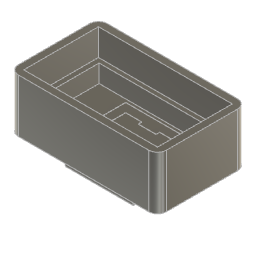
Master Arm AA AG v11 (Autodesk Fusion 360 design; units mm, degrees)
Autodesk Fusion 360 part; units mm, degrees
(part 1 of 6)
sketch "Master Arm Legend Plate" plane through (-25, -275, 0) normal (0, 0, 1) x (1, 0, 0)
  line L0 (41.275, 261.179028) -> (41.521944, 261.14375)
  line L1 (42.545, 261.955139) -> (42.545, 262.202083)
  line L2 (41.521944, 261.14375) -> (41.839444, 261.179028)
  line L3 (8.678333, 226.924305) -> (8.713611, 226.994861)
  line L4 (8.713611, 226.994861) -> (8.748889, 227.100694)
  line L5 (6.385278, 226.85375) -> (8.396111, 226.85375)
  line L6 (32.984722, 286.190972) -> (33.196389, 286.120417)
  line L7 (33.196389, 286.120417) -> (33.443333, 286.085139)
  line L8 (42.051111, 264.424583) -> (41.874722, 264.671528)
  line L9 (23.459722, 289.295417) -> (21.448889, 289.295417)
  line L10 (21.448889, 289.295417) -> (21.448889, 288.201805)
  line L11 (21.448889, 288.201805) -> (22.895278, 288.201805)
  line L12 (37.958889, 291.059305) -> (35.771667, 291.059305)
  line L13 (35.595278, 285.555972) -> (35.489444, 285.59125)
  line L14 (31.220833, 295.222083) -> (31.291389, 295.11625)
  line L15 (30.056667, 253.594305) -> (30.127222, 253.594305)
  line L16 (35.771667, 227.241805) -> (35.771667, 227.100694)
  line L17 (43.991389, 295.821805) -> (43.991389, 295.186805)
  line L18 (25.646944, 224.878194) -> (25.752778, 224.984028)
  line L19 (42.721389, 272.503194) -> (42.721389, 272.397361)
  line L20 (42.721389, 272.397361) -> (42.686111, 272.326805)
  line L21 (42.686111, 272.326805) -> (42.580278, 272.25625)
  line L22 (42.580278, 272.25625) -> (42.474444, 272.25625)
  line L23 (42.474444, 272.25625) -> (42.403889, 272.25625)
  line L24 (42.403889, 272.25625) -> (42.333333, 272.291528)
  line L25 (42.333333, 272.291528) -> (42.262778, 272.362083)
  line L26 (42.262778, 272.362083) -> (42.2275, 272.432639)
  line L27 (42.2275, 272.432639) -> (42.051111, 272.961805)
  line L28 (42.051111, 272.961805) -> (40.604722, 272.961805)
  line L29 (40.604722, 272.961805) -> (40.463611, 272.397361)
  line L30 (40.463611, 272.397361) -> (40.428333, 272.326805)
  line L31 (40.428333, 272.326805) -> (40.393056, 272.291528)
  line L32 (40.393056, 272.291528) -> (40.287222, 272.25625)
  line L33 (40.287222, 272.25625) -> (40.216667, 272.25625)
  line L34 (40.216667, 272.25625) -> (40.040278, 272.291528)
  line L35 (40.040278, 272.291528) -> (39.969722, 272.362083)
  line L36 (39.969722, 272.362083) -> (39.934444, 272.467917)
  line L37 (39.934444, 272.467917) -> (39.969722, 272.57375)
  line L38 (39.969722, 272.57375) -> (40.005, 272.679583)
  line L39 (40.005, 272.679583) -> (41.063333, 276.313194)
  line L40 (41.063333, 276.313194) -> (41.098611, 276.38375)
  line L41 (41.098611, 276.38375) -> (41.133889, 276.454305)
  line L42 (41.133889, 276.454305) -> (41.239722, 276.489583)
  line L43 (41.239722, 276.489583) -> (41.345556, 276.489583)
  line L44 (41.345556, 276.489583) -> (41.416111, 276.489583)
  line L45 (41.416111, 276.489583) -> (41.486667, 276.454305)
  line L46 (41.486667, 276.454305) -> (41.557222, 276.348472)
  line L47 (41.557222, 276.348472) -> (41.5925, 276.242639)
  line L48 (41.5925, 276.242639) -> (42.686111, 272.644305)
  line L49 (42.686111, 272.644305) -> (42.721389, 272.57375)
  line L50 (42.721389, 272.57375) -> (42.721389, 272.503194)
  line L51 (33.196389, 241.14125) -> (33.161111, 241.77625)
  line L52 (33.161111, 241.77625) -> (33.090556, 242.375972)
  line L53 (33.090556, 242.375972) -> (32.949444, 243.010972)
  line L54 (32.949444, 243.010972) -> (32.737778, 243.575417)
  line L55 (32.737778, 243.575417) -> (32.455556, 244.139861)
  line L56 (32.455556, 244.139861) -> (32.138056, 244.669028)
  line L57 (32.138056, 244.669028) -> (31.75, 245.198194)
  line L58 (31.75, 245.198194) -> (31.361944, 245.656805)
  line L59 (31.361944, 245.656805) -> (30.868056, 246.080139)
  line L60 (30.868056, 246.080139) -> (30.374167, 246.432917)
  line L61 (30.374167, 246.432917) -> (29.845, 246.750417)
  line L62 (29.845, 246.750417) -> (29.280556, 247.032639)
  line L63 (29.280556, 247.032639) -> (28.716111, 247.244305)
  line L64 (28.716111, 247.244305) -> (28.081111, 247.385417)
  line L65 (28.081111, 247.385417) -> (27.481389, 247.455972)
  line L66 (27.481389, 247.455972) -> (26.846389, 247.49125)
  line L67 (26.846389, 247.49125) -> (26.246667, 247.455972)
  line L68 (26.246667, 247.455972) -> (25.611667, 247.385417)
  line L69 (25.611667, 247.385417) -> (25.011944, 247.244305)
  line L70 (25.011944, 247.244305) -> (24.412222, 247.032639)
  line L71 (24.412222, 247.032639) -> (23.847778, 246.750417)
  line L72 (23.847778, 246.750417) -> (23.318611, 246.432917)
  line L73 (23.318611, 246.432917) -> (22.824722, 246.080139)
  line L74 (22.824722, 246.080139) -> (22.366111, 245.656805)
  line L75 (22.366111, 245.656805) -> (21.942778, 245.198194)
  line L76 (21.942778, 245.198194) -> (21.59, 244.669028)
  line L77 (21.59, 244.669028) -> (21.2725, 244.139861)
  line L78 (21.2725, 244.139861) -> (20.990278, 243.575417)
  line L79 (20.990278, 243.575417) -> (20.778611, 243.010972)
  line L80 (20.778611, 243.010972) -> (20.6375, 242.375972)
  line L81 (20.6375, 242.375972) -> (20.531667, 241.77625)
  line L82 (20.531667, 241.77625) -> (20.496389, 241.14125)
  line L83 (20.496389, 241.14125) -> (20.531667, 240.541528)
  line L84 (20.531667, 240.541528) -> (20.6375, 239.906528)
  line L85 (20.6375, 239.906528) -> (20.778611, 239.306805)
  line L86 (20.778611, 239.306805) -> (20.990278, 238.707083)
  line L87 (20.990278, 238.707083) -> (21.2725, 238.177917)
  line L88 (21.2725, 238.177917) -> (21.59, 237.613472)
  line L89 (21.59, 237.613472) -> (21.942778, 237.119583)
  line L90 (21.942778, 237.119583) -> (22.366111, 236.660972)
  line L91 (22.366111, 236.660972) -> (22.824722, 236.237639)
  line L92 (22.824722, 236.237639) -> (23.318611, 235.884861)
  line L93 (23.318611, 235.884861) -> (23.847778, 235.567361)
  line L94 (23.847778, 235.567361) -> (24.412222, 235.285139)
  line L95 (24.412222, 235.285139) -> (25.011944, 235.073472)
  line L96 (25.011944, 235.073472) -> (25.611667, 234.932361)
  line L97 (25.611667, 234.932361) -> (26.246667, 234.826528)
  line L98 (26.246667, 234.826528) -> (26.846389, 234.79125)
  line L99 (26.846389, 234.79125) -> (27.481389, 234.826528)
  line L100 (27.481389, 234.826528) -> (28.081111, 234.932361)
  line L101 (28.081111, 234.932361) -> (28.716111, 235.073472)
  line L102 (28.716111, 235.073472) -> (29.280556, 235.285139)
  line L103 (29.280556, 235.285139) -> (29.845, 235.567361)
  line L104 (29.845, 235.567361) -> (30.374167, 235.884861)
  line L105 (30.374167, 235.884861) -> (30.868056, 236.237639)
  line L106 (30.868056, 236.237639) -> (31.361944, 236.660972)
  line L107 (31.361944, 236.660972) -> (31.75, 237.119583)
  line L108 (31.75, 237.119583) -> (32.138056, 237.613472)
  line L109 (32.138056, 237.613472) -> (32.455556, 238.177917)
  line L110 (32.455556, 238.177917) -> (32.737778, 238.707083)
  line L111 (32.737778, 238.707083) -> (32.949444, 239.306805)
  line L112 (32.949444, 239.306805) -> (33.090556, 239.906528)
  line L113 (33.090556, 239.906528) -> (33.161111, 240.541528)
  line L114 (33.161111, 240.541528) -> (33.196389, 241.14125)
  line L115 (33.831389, 294.728194) -> (34.043056, 294.587083)
  line L116 (10.089444, 235.602639) -> (10.442222, 235.461528)
  line L117 (10.442222, 235.461528) -> (10.724444, 235.249861)
  line L118 (30.868056, 230.381528) -> (30.938611, 230.381528)
  line L119 (30.938611, 230.381528) -> (31.044444, 230.416805)
  line L120 (31.044444, 230.416805) -> (31.079722, 230.416805)
  line L121 (21.942778, 225.513194) -> (22.013333, 225.548472)
  line L122 (18.273889, 226.85375) -> (18.485556, 226.85375)
  line L123 (18.485556, 226.85375) -> (18.626667, 226.783194)
  line L124 (38.4175, 253.20625) -> (38.452778, 253.170972)
  line L125 (32.490833, 291.165139) -> (32.526111, 291.376805)
  line L126 (20.919722, 285.90875) -> (20.919722, 289.471805)
  line L127 (20.919722, 289.471805) -> (20.919722, 289.612917)
  line L128 (20.919722, 289.612917) -> (20.955, 289.71875)
  line L129 (41.733611, 263.542639) -> (41.627778, 263.542639)
  line L130 (41.627778, 263.542639) -> (41.521944, 263.507361)
  line L131 (40.040278, 253.100417) -> (40.110833, 253.170972)
  line L132 (41.980556, 265.27125) -> (42.192222, 265.130139)
  line L133 (42.509722, 264.354028) -> (42.403889, 264.283472)
  line L134 (41.768889, 261.708194) -> (41.874722, 261.77875)
  line L135 (39.828611, 231.404583) -> (39.793333, 231.686805)
  line L136 (39.793333, 231.686805) -> (39.722778, 231.863194)
  line L137 (39.722778, 231.863194) -> (39.581667, 231.969028)
  line L138 (39.581667, 231.969028) -> (39.511111, 232.039583)
  line L139 (39.511111, 232.039583) -> (39.37, 232.039583)
  line L140 (39.37, 232.039583) -> (38.735, 232.039583)
  line L141 (38.735, 232.039583) -> (38.735, 230.769583)
  line L142 (38.735, 230.769583) -> (39.334722, 230.769583)
  line L143 (39.334722, 230.769583) -> (39.475833, 230.769583)
  line L144 (39.475833, 230.769583) -> (39.581667, 230.840139)
  line L145 (39.581667, 230.840139) -> (39.652222, 230.910694)
  line L146 (39.652222, 230.910694) -> (39.793333, 231.087083)
  line L147 (39.793333, 231.087083) -> (39.828611, 231.404583)
  line L148 (42.474444, 263.507361) -> (42.545, 263.36625)
  line L149 (14.2875, 290.177361) -> (14.075833, 289.824583)
  line L150 (14.075833, 289.824583) -> (13.97, 289.471805)
  line L151 (9.913056, 223.255417) -> (9.877778, 223.220139)
  line L152 (38.946667, 276.807083) -> (39.017222, 276.807083)
  line L153 (34.572222, 289.189583) -> (34.6075, 289.08375)
  line L154 (34.6075, 289.08375) -> (34.642778, 288.977917)
  line L155 (21.131389, 285.555972) -> (21.025556, 285.626528)
  line L156 (21.025556, 285.626528) -> (20.919722, 285.767639)
  line L157 (20.919722, 285.767639) -> (20.919722, 285.90875)
  line L158 (31.361944, 245.656805) -> (30.868056, 246.080139)
  line L159 (30.868056, 246.080139) -> (30.374167, 246.432917)
  line L160 (41.310278, 261.708194) -> (41.557222, 261.672917)
  line L161 (25.893889, 225.019305) -> (26.035, 224.984028)
  line L162 (42.721389, 272.397361) -> (42.721389, 272.503194)
  line L163 (35.806944, 261.320139) -> (35.842222, 261.249583)
  line L164 (38.311667, 244.245694) -> (38.276389, 243.928194)
  line L165 (34.536944, 291.059305) -> (34.642778, 291.094583)
  line L166 (31.291389, 295.010417) -> (31.291389, 291.341528)
  line L167 (32.243889, 279.135417) -> (32.208611, 279.452917)
  line L168 (28.363333, 223.714028) -> (28.575, 224.066805)
  line L169 (25.611667, 224.63125) -> (25.682222, 224.207917)
  line L170 (25.682222, 224.207917) -> (25.893889, 223.784583)
  line L171 (32.102778, 245.939028) -> (31.644167, 246.397639)
  line L172 (31.644167, 246.397639) -> (31.150278, 246.820972)
  line L173 (42.474444, 264.777361) -> (42.580278, 264.565694)
  line L174 (31.115, 230.557917) -> (31.115, 230.628472)
  line L175 (28.716111, 230.452083) -> (28.716111, 230.557917)
  line L176 (27.6225, 230.381528) -> (28.433889, 230.381528)
  line L177 (27.6225, 228.970417) -> (27.6225, 230.381528)
  line L178 (14.851944, 290.741805) -> (14.534444, 290.494861)
  line L179 (14.534444, 290.494861) -> (14.2875, 290.177361)
  line L180 (21.2725, 244.139861) -> (21.59, 244.669028)
  line L181 (27.269722, 294.939861) -> (27.305, 295.080972)
  line L182 (24.765, 289.471805) -> (24.729722, 289.577639)
  line L183 (39.123056, 265.694583) -> (39.0525, 265.624028)
  line L184 (24.729722, 289.577639) -> (24.765, 289.648194)
  line L185 (32.490833, 286.755417) -> (32.7025, 286.437917)
  line L186 (32.7025, 286.437917) -> (32.984722, 286.190972)
  line L187 (38.241111, 236.555139) -> (38.382222, 236.625694)
  line L188 (40.3225, 236.308194) -> (40.287222, 236.237639)
  line L189 (38.4175, 228.75875) -> (38.488056, 228.723472)
  line L190 (38.276389, 229.040972) -> (38.276389, 228.899861)
  line L191 (19.05, 226.148194) -> (19.014722, 226.324583)
  line L192 (19.014722, 226.324583) -> (18.944167, 226.500972)
  line L193 (18.944167, 226.500972) -> (18.803056, 226.677361)
  line L194 (18.803056, 226.677361) -> (18.626667, 226.783194)
  line L195 (18.626667, 226.783194) -> (18.485556, 226.85375)
  line L196 (18.485556, 226.85375) -> (18.273889, 226.85375)
  line L197 (18.273889, 226.85375) -> (17.321389, 226.85375)
  line L198 (17.321389, 226.85375) -> (17.321389, 225.407361)
  line L199 (17.321389, 225.407361) -> (18.238611, 225.407361)
  line L200 (18.238611, 225.407361) -> (18.415, 225.442639)
  line L201 (18.415, 225.442639) -> (18.626667, 225.477917)
  line L202 (18.626667, 225.477917) -> (18.803056, 225.58375)
  line L203 (18.803056, 225.58375) -> (18.908889, 225.724861)
  line L204 (18.908889, 225.724861) -> (19.014722, 225.936528)
  line L205 (19.014722, 225.936528) -> (19.05, 226.148194)
  line L206 (38.664444, 236.167083) -> (40.040278, 236.167083)
  line L207 (38.664444, 235.214583) -> (38.664444, 236.167083)
  line L208 (39.6875, 235.214583) -> (38.664444, 235.214583)
  line L209 (39.934444, 235.002917) -> (39.934444, 235.073472)
  line L210 (21.942778, 225.019305) -> (21.872222, 225.054583)
  line L211 (38.735, 243.928194) -> (38.770278, 243.751805)
  line L212 (34.642778, 287.637361) -> (34.642778, 286.614305)
  line L213 (34.642778, 286.614305) -> (34.6075, 286.367361)
  line L214 (39.0525, 227.382917) -> (39.264167, 227.312361)
  line L215 (39.264167, 227.312361) -> (39.37, 227.241805)
  line L216 (39.228889, 276.419028) -> (39.193611, 276.277917)
  line L217 (27.481389, 232.004305) -> (28.821944, 232.004305)
  line L218 (33.760833, 285.626528) -> (33.408056, 285.555972)
  line L219 (33.408056, 285.555972) -> (33.090556, 285.59125)
  line L220 (29.598056, 293.422917) -> (29.562778, 293.317083)
  line L221 (30.021389, 250.313472) -> (29.986111, 250.34875)
  line L222 (26.246667, 247.455972) -> (26.846389, 247.49125)
  line L223 (26.176111, 223.467083) -> (25.893889, 223.784583)
  line L224 (16.792222, 286.931805) -> (17.109722, 287.108194)
  line L225 (17.109722, 287.108194) -> (17.427222, 287.284583)
  line L226 (37.817778, 287.707917) -> (35.806944, 287.707917)
  line L227 (43.991389, 287.390417) -> (43.991389, 282.486805)
  line L228 (20.531667, 240.541528) -> (20.496389, 241.14125)
  line L229 (37.641389, 293.21125) -> (37.394444, 293.175972)
  line L230 (40.428333, 272.326805) -> (40.463611, 272.397361)
  line L231 (39.934444, 272.467917) -> (39.969722, 272.362083)
  line L232 (39.698083, 284.522333) -> (39.334722, 284.885694)
  line L233 (39.405278, 265.624028) -> (39.440556, 265.553472)
  line L234 (40.357778, 240.541528) -> (40.3225, 240.470972)
  line L235 (33.196389, 226.85375) -> (32.984722, 226.889028)
  line L236 (32.984722, 226.889028) -> (32.914167, 226.959583)
  line L237 (9.595556, 227.347639) -> (9.666111, 227.347639)
  line L238 (33.478611, 243.716528) -> (33.231667, 244.31625)
  line L239 (33.231667, 244.31625) -> (32.914167, 244.880694)
  line L240 (37.076944, 272.25625) -> (36.971111, 272.25625)
  line L241 (26.846389, 247.49125) -> (27.481389, 247.455972)
  line L242 (34.360556, 288.695694) -> (34.29, 288.695694)
  line L243 (34.29, 288.695694) -> (34.219444, 288.730972)
  line L244 (30.303611, 250.454583) -> (30.303611, 250.384028)
  line L245 (14.781389, 280.722917) -> (30.656389, 280.722917)
  line L246 (33.831389, 242.446528) -> (33.690278, 243.116805)
  line L247 (33.690278, 243.116805) -> (33.478611, 243.716528)
  line L248 (30.338889, 250.525139) -> (30.303611, 250.454583)
  line L249 (39.264167, 276.665972) -> (39.264167, 276.524861)
  line L250 (34.29, 287.990139) -> (33.655, 287.990139)
  line L251 (40.216667, 249.431528) -> (40.146111, 249.466805)
  line L252 (29.986111, 229.111528) -> (29.986111, 230.381528)
  line L253 (23.106944, 225.336805) -> (23.106944, 225.195694)
  line L254 (14.005278, 288.307639) -> (14.181667, 287.954861)
  line L255 (14.181667, 287.954861) -> (14.393333, 287.637361)
  line L256 (29.598056, 231.757361) -> (29.598056, 231.827917)
  line L257 (22.577778, 235.461528) -> (23.106944, 235.10875)
  line L258 (23.106944, 235.10875) -> (23.671389, 234.79125)
  line L259 (25.893889, 223.784583) -> (25.682222, 224.207917)
  line L260 (28.645556, 224.419583) -> (28.575, 224.066805)
  line L261 (29.562778, 293.317083) -> (29.5275, 293.246528)
  line L262 (37.218056, 272.291528) -> (37.1475, 272.25625)
  line L263 (30.691667, 289.295417) -> (29.845, 289.295417)
  line L264 (32.596667, 288.695694) -> (32.349722, 288.272361)
  line L265 (32.349722, 288.272361) -> (32.279167, 287.990139)
  line L266 (38.241111, 289.71875) -> (38.205833, 289.754028)
  line L267 (38.205833, 289.754028) -> (38.170556, 289.789305)
  line L268 (23.671389, 234.79125) -> (24.271111, 234.509028)
  line L269 (24.271111, 234.509028) -> (24.906111, 234.297361)
  line L270 (36.900556, 272.291528) -> (36.83, 272.397361)
  line L271 (40.357778, 249.466805) -> (40.216667, 249.431528)
  line L272 (27.305, 295.080972) -> (27.340278, 295.186805)
  line L273 (35.806944, 295.292639) -> (37.994167, 295.292639)
  line L274 (37.1475, 272.25625) -> (37.076944, 272.25625)
  line L275 (38.664444, 234.755972) -> (38.664444, 233.344861)
  line L276 (36.971111, 272.25625) -> (36.900556, 272.291528)
  line L277 (34.642778, 287.637361) -> (34.6075, 287.778472)
  line L278 (34.6075, 287.778472) -> (34.536944, 287.919583)
  line L279 (32.984722, 289.154305) -> (32.773056, 288.942639)
  line L280 (32.773056, 288.942639) -> (32.596667, 288.695694)
  line L281 (36.865278, 272.679583) -> (36.865278, 272.714861)
  line L282 (29.421667, 223.184861) -> (29.351111, 223.325972)
  line L283 (39.087778, 237.084305) -> (39.158333, 237.01375)
  line L284 (39.158333, 237.01375) -> (39.264167, 237.01375)
  line L285 (27.551944, 291.059305) -> (27.6225, 291.059305)
  line L286 (16.016111, 223.149583) -> (15.769167, 223.114305)
  line L287 (30.197778, 253.594305) -> (30.268333, 253.559028)
  line L288 (15.980833, 223.643472) -> (15.875, 223.643472)
  line L289 (15.875, 223.643472) -> (15.804444, 223.643472)
  line L290 (29.845, 246.750417) -> (30.374167, 246.432917)
  line L291 (25.611667, 224.63125) -> (25.611667, 224.737083)
  line L292 (27.199167, 231.722083) -> (27.199167, 231.827917)
  line L293 (1.446389, 284.709305) -> (5.150556, 292.999583)
  line L294 (42.580278, 264.565694) -> (42.474444, 264.777361)
  line L295 (19.755556, 241.14125) -> (19.790833, 240.50625)
  line L296 (19.790833, 240.50625) -> (19.861389, 239.835972)
  line L297 (39.581667, 244.422083) -> (39.37, 244.457361)
  line L298 (27.798889, 291.30625) -> (27.798889, 291.200417)
  line L299 (15.769167, 223.114305) -> (16.016111, 223.149583)
  line L300 (40.146111, 244.457361) -> (40.216667, 244.280972)
  line L301 (23.106944, 226.465694) -> (23.106944, 226.53625)
  line L302 (22.577778, 226.430417) -> (22.718889, 226.289305)
  line L303 (22.718889, 226.289305) -> (22.789444, 226.254028)
  line L304 (31.608889, 225.689583) -> (31.644167, 225.58375)
  line L305 (25.153056, 289.754028) -> (25.294167, 289.612917)
  line L306 (31.291389, 280.581805) -> (31.538333, 280.440694)
  line L307 (27.305, 252.88875) -> (27.340278, 252.641805)
  line L308 (8.748889, 227.100694) -> (8.713611, 227.206528)
  line L309 (8.713611, 227.206528) -> (8.678333, 227.277083)
  line L310 (8.678333, 227.277083) -> (8.607778, 227.347639)
  line L311 (29.739167, 228.723472) -> (29.845, 228.723472)
  line L312 (29.598056, 231.757361) -> (29.598056, 228.970417)
  line L313 (29.845, 232.004305) -> (29.739167, 232.004305)
  line L314 (28.716111, 230.628472) -> (28.716111, 230.557917)
  line L315 (35.277778, 273.490972) -> (34.148889, 273.490972)
  line L316 (34.148889, 273.490972) -> (34.713333, 275.325417)
  line L317 (21.59, 244.669028) -> (21.2725, 244.139861)
  line L318 (21.2725, 244.139861) -> (20.990278, 243.575417)
  line L319 (30.868056, 236.237639) -> (30.374167, 235.884861)
  line L320 (9.595556, 227.347639) -> (9.489722, 227.312361)
  line L321 (9.489722, 227.312361) -> (9.454444, 227.241805)
  line L322 (32.173333, 223.537639) -> (32.208611, 223.467083)
  line L323 (33.372778, 287.919583) -> (33.443333, 287.954861)
  line L324 (33.443333, 287.954861) -> (33.549167, 287.990139)
  line L325 (14.322778, 295.821805) -> (19.261667, 295.821805)
  line L326 (17.885833, 281.745972) -> (12.946944, 281.745972)
  line L327 (32.102778, 226.889028) -> (31.996944, 226.85375)
  line L328 (36.583056, 227.312361) -> (36.83, 227.382917)
  line L329 (29.351111, 223.325972) -> (29.315833, 223.467083)
  line L330 (34.219444, 294.234305) -> (34.254722, 294.057917)
  line L331 (33.196389, 241.14125) -> (33.161111, 240.541528)
  line L332 (31.785278, 257.369028) -> (31.538333, 257.157361)
  line L333 (18.626667, 225.477917) -> (18.415, 225.442639)
  line L334 (10.442222, 235.461528) -> (10.089444, 235.602639)
  line L335 (10.089444, 235.602639) -> (9.736667, 235.673194)
  line L336 (9.736667, 235.673194) -> (9.383889, 235.673194)
  line L337 (23.847778, 235.567361) -> (23.318611, 235.884861)
  line L338 (33.161111, 241.77625) -> (33.196389, 241.14125)
  line L339 (37.711944, 293.599305) -> (37.747222, 293.52875)
  line L340 (32.949444, 239.306805) -> (32.737778, 238.707083)
  line L341 (31.467778, 231.722083) -> (31.397222, 231.651528)
  line L342 (34.819167, 265.377083) -> (34.748611, 265.341805)
  line L343 (34.748611, 265.341805) -> (34.678056, 265.27125)
  line L344 (34.678056, 265.27125) -> (34.642778, 265.200694)
  line L345 (39.334722, 295.43375) -> (39.334722, 295.821805)
  line L346 (27.375556, 286.014583) -> (27.446111, 285.944028)
  line L347 (31.891111, 223.643472) -> (31.961667, 223.643472)
  line L348 (38.558611, 249.749028) -> (38.523333, 249.537361)
  line L349 (36.935833, 281.745972) -> (39.698083, 284.522333)
  line L350 (22.013333, 225.019305) -> (22.119167, 225.019305)
  line L351 (38.981944, 265.553472) -> (37.076944, 261.602361)
  line L352 (39.228889, 265.694583) -> (39.123056, 265.694583)
  line L353 (40.463611, 252.959305) -> (40.463611, 253.100417)
  line L354 (40.463611, 253.100417) -> (40.393056, 253.170972)
  line L355 (40.393056, 253.170972) -> (40.3225, 253.20625)
  line L356 (16.016111, 226.889028) -> (16.051389, 226.924305)
  line L357 (28.539722, 227.347639) -> (28.610278, 227.312361)
  line L358 (42.439167, 261.637639) -> (42.545, 261.955139)
  line L359 (29.280556, 251.442361) -> (29.245278, 251.442361)
  line L360 (40.005, 251.93625) -> (39.511111, 250.913194)
  line L361 (18.415, 225.442639) -> (18.238611, 225.407361)
  line L362 (18.626667, 226.783194) -> (18.803056, 226.677361)
  line L363 (8.748889, 223.255417) -> (8.713611, 223.220139)
  line L364 (8.713611, 223.220139) -> (8.643056, 223.149583)
  line L365 (11.006667, 235.038194) -> (10.724444, 235.249861)
  line L366 (10.724444, 235.249861) -> (10.442222, 235.461528)
  line L367 (31.644167, 225.513194) -> (31.608889, 225.372083)
  line L368 (37.676667, 223.396528) -> (37.676667, 223.290694)
  line L369 (37.676667, 226.85375) -> (37.676667, 223.467083)
  line L370 (36.794722, 226.85375) -> (37.676667, 226.85375)
  line L371 (22.154444, 226.818472) -> (22.330833, 226.712639)
  line L372 (22.330833, 226.712639) -> (22.577778, 226.430417)
  line L373 (21.060833, 226.254028) -> (21.237222, 226.500972)
  line L374 (15.522222, 225.689583) -> (15.451667, 225.724861)
  line L375 (15.451667, 225.724861) -> (15.24, 225.760139)
  line L376 (15.204722, 225.26625) -> (15.451667, 225.301528)
  line L377 (29.280556, 235.285139) -> (28.716111, 235.073472)
  line L378 (38.276389, 241.740972) -> (38.205833, 242.164305)
  line L379 (26.740556, 289.754028) -> (26.67, 289.648194)
  line L380 (27.199167, 253.559028) -> (26.916944, 253.594305)
  line L381 (28.645556, 253.488472) -> (28.610278, 253.52375)
  line L382 (43.074167, 218.034306) -> (43.991389, 218.034306)
  line L383 (29.950833, 222.549861) -> (25.435278, 218.034306)
  line L384 (40.781111, 262.590139) -> (40.675278, 262.907639)
  line L385 (30.021389, 234.79125) -> (30.585833, 235.10875)
  line L386 (30.585833, 235.10875) -> (31.150278, 235.461528)
  line L387 (43.991389, 293.740417) -> (43.991389, 288.836805)
  line L388 (32.208611, 289.119028) -> (31.926389, 288.589861)
  line L389 (25.964444, 250.595694) -> (25.964444, 250.454583)
  line L390 (25.964444, 250.454583) -> (25.964444, 250.419305)
  line L391 (16.157222, 223.396528) -> (16.121944, 223.467083)
  line L392 (16.121944, 223.467083) -> (16.086667, 223.537639)
  line L393 (16.086667, 223.537639) -> (15.980833, 223.643472)
  line L394 (39.123056, 241.14125) -> (38.770278, 241.211805)
  line L395 (24.412222, 247.032639) -> (25.011944, 247.244305)
  line L396 (31.785278, 288.13125) -> (31.926389, 288.589861)
  line L397 (31.926389, 288.589861) -> (32.208611, 289.119028)
  line L398 (34.642778, 291.094583) -> (34.748611, 291.165139)
  line L399 (39.334722, 289.08375) -> (43.991389, 293.740417)
  line L400 (24.800278, 289.365972) -> (24.765, 289.471805)
  line L401 (37.747222, 293.317083) -> (37.711944, 293.246528)
  line L402 (27.163889, 289.683472) -> (27.093333, 289.754028)
  line L403 (28.328056, 250.34875) -> (28.292778, 250.384028)
  line L404 (23.318611, 235.884861) -> (22.824722, 236.237639)
  line L405 (35.136667, 265.235972) -> (35.066111, 265.341805)
  line L406 (35.066111, 265.341805) -> (34.995556, 265.377083)
  line L407 (9.383889, 235.673194) -> (9.736667, 235.673194)
  line L408 (9.736667, 235.673194) -> (10.089444, 235.602639)
  line L409 (12.206111, 223.149583) -> (12.135556, 223.184861)
  line L410 (40.781111, 273.490972) -> (41.345556, 275.325417)
  line L411 (24.341667, 252.677083) -> (24.765, 251.265972)
  line L412 (21.872222, 225.054583) -> (21.942778, 225.019305)
  line L413 (21.942778, 225.019305) -> (22.013333, 225.019305)
  line L414 (31.220833, 231.61625) -> (31.326667, 231.61625)
  line L415 (22.965833, 226.289305) -> (22.86, 226.254028)
  line L416 (25.435278, 250.489861) -> (25.435278, 250.560417)
  line L417 (33.513889, 261.355417) -> (33.549167, 261.249583)
  line L418 (13.6525, 280.264305) -> (13.476111, 280.017361)
  line L419 (27.798889, 293.175972) -> (29.21, 293.175972)
  line L420 (27.798889, 291.376805) -> (27.798889, 293.175972)
  line L421 (27.798889, 291.200417) -> (27.798889, 291.30625)
  line L422 (27.798889, 291.30625) -> (27.798889, 291.376805)
  line L423 (28.821944, 231.61625) -> (27.6225, 231.61625)
  line L424 (25.646944, 233.380139) -> (26.317222, 233.309583)
  line L425 (26.317222, 233.309583) -> (27.022778, 233.274305)
  line L426 (27.022778, 233.274305) -> (27.728333, 233.344861)
  line L427 (27.728333, 233.344861) -> (28.398611, 233.450694)
  line L428 (26.3525, 228.723472) -> (26.387778, 228.723472)
  line L429 (26.387778, 228.723472) -> (26.458333, 228.723472)
  line L430 (34.536944, 276.454305) -> (34.466389, 276.38375)
  line L431 (34.466389, 276.38375) -> (34.466389, 276.313194)
  line L432 (29.421667, 251.477639) -> (29.351111, 251.442361)
  line L433 (21.801667, 225.125139) -> (21.766389, 225.26625)
  line L434 (38.664444, 242.199583) -> (38.664444, 241.987917)
  line L435 (23.953611, 229.323194) -> (23.988889, 229.640694)
  line L436 (22.895278, 228.688194) -> (23.142222, 228.723472)
  line L437 (42.545, 264.459861) -> (42.580278, 264.565694)
  line L438 (28.433889, 230.381528) -> (28.645556, 230.381528)
  line L439 (28.645556, 230.381528) -> (28.680833, 230.416805)
  line L440 (28.680833, 230.416805) -> (28.716111, 230.452083)
  line L441 (25.646944, 281.745972) -> (28.786667, 284.885694)
  line L442 (34.572222, 226.85375) -> (34.572222, 223.431805)
  line L443 (37.817778, 289.648194) -> (37.853056, 289.71875)
  line L444 (22.895278, 231.61625) -> (23.106944, 231.61625)
  line L445 (22.718889, 231.545694) -> (22.824722, 231.580972)
  line L446 (39.334722, 284.885694) -> (39.334722, 289.08375)
  line L447 (30.585833, 281.745972) -> (25.646944, 281.745972)
  line L448 (22.119167, 229.746528) -> (22.083889, 229.570139)
  line L449 (22.507222, 229.605417) -> (22.471944, 229.71125)
  line L450 (22.789444, 226.254028) -> (22.86, 226.254028)
  line L451 (21.9075, 226.85375) -> (22.154444, 226.818472)
  line L452 (29.421667, 293.21125) -> (29.5275, 293.246528)
  line L453 (29.5275, 293.246528) -> (29.562778, 293.317083)
  line L454 (29.562778, 293.317083) -> (29.598056, 293.422917)
  line L455 (29.21, 293.175972) -> (29.351111, 293.175972)
  line L456 (35.418889, 289.754028) -> (35.489444, 289.789305)
  line L457 (26.176111, 224.63125) -> (26.211389, 224.31375)
  line L458 (32.279167, 291.059305) -> (32.385, 291.059305)
  line L459 (29.915556, 252.465417) -> (29.915556, 250.560417)
  line L460 (29.492222, 251.583472) -> (29.915556, 252.465417)
  line L461 (21.766389, 225.26625) -> (21.801667, 225.407361)
  line L462 (29.915556, 250.560417) -> (29.915556, 250.454583)
  line L463 (29.915556, 250.454583) -> (29.950833, 250.384028)
  line L464 (12.065, 223.431805) -> (12.065, 226.112917)
  line L465 (40.075556, 233.344861) -> (40.251944, 233.309583)
  line L466 (33.090556, 285.59125) -> (33.408056, 285.555972)
  line L467 (31.75, 287.672639) -> (31.785278, 287.249305)
  line L468 (28.645556, 253.488472) -> (29.280556, 252.112639)
  line L469 (28.539722, 253.594305) -> (28.575, 253.559028)
  line L470 (28.610278, 253.52375) -> (28.575, 253.559028)
  line L471 (28.575, 253.559028) -> (28.539722, 253.594305)
  line L472 (13.899444, 289.048472) -> (13.934722, 288.695694)
  line L473 (33.513889, 287.460972) -> (33.478611, 287.460972)
  line L474 (33.478611, 287.460972) -> (33.408056, 287.49625)
  line L475 (23.318611, 246.432917) -> (22.824722, 246.080139)
  line L476 (22.824722, 246.080139) -> (22.366111, 245.656805)
  line L477 (29.104167, 233.591805) -> (29.739167, 233.83875)
  line L478 (29.739167, 233.83875) -> (30.374167, 234.120972)
  line L479 (30.374167, 234.120972) -> (31.009167, 234.438472)
  line L480 (33.372778, 287.919583) -> (33.3375, 287.849028)
  line L481 (33.3375, 287.849028) -> (33.302222, 287.707917)
  line L482 (31.855833, 226.85375) -> (29.845, 226.85375)
  line L483 (40.534167, 264.671528) -> (40.287222, 264.142361)
  line L484 (40.287222, 264.142361) -> (40.181389, 263.719028)
  line L485 (40.181389, 263.719028) -> (40.146111, 263.260417)
  line L486 (41.521944, 265.377083) -> (41.133889, 265.306528)
  line L487 (37.006389, 261.390694) -> (37.006389, 261.46125)
  line L488 (27.446111, 251.865694) -> (27.6225, 252.147917)
  line L489 (27.6225, 252.147917) -> (27.728333, 252.394861)
  line L490 (27.728333, 252.394861) -> (27.763611, 252.641805)
  line L491 (38.276389, 289.612917) -> (38.276389, 289.507083)
  line L492 (9.666111, 227.347639) -> (9.736667, 227.347639)
  line L493 (35.983333, 291.588472) -> (35.983333, 293.175972)
  line L494 (37.994167, 291.588472) -> (35.983333, 291.588472)
  line L495 (38.170556, 291.553194) -> (38.064722, 291.553194)
  line L496 (12.347222, 227.382917) -> (12.453056, 227.347639)
  line L497 (17.885833, 281.745972) -> (21.025556, 284.885694)
  line L498 (43.991389, 282.486805) -> (43.991389, 287.390417)
  line L499 (29.139444, 251.512917) -> (29.174722, 251.442361)
  line L500 (29.174722, 251.442361) -> (29.245278, 251.442361)
  line L501 (28.786667, 284.885694) -> (33.725556, 284.885694)
  line L502 (34.184167, 294.410694) -> (34.219444, 294.234305)
  line L503 (35.348333, 289.577639) -> (35.348333, 289.648194)
  line L504 (1.446389, 281.745972) -> (1.446389, 282.945417)
  line L505 (23.106944, 226.53625) -> (23.106944, 226.465694)
  line L506 (40.005, 249.607917) -> (40.005, 249.71375)
  line L507 (26.105556, 224.94875) -> (26.140833, 224.878194)
  line L508 (38.205833, 285.626528) -> (38.170556, 285.59125)
  line L509 (27.551944, 291.059305) -> (27.410833, 291.094583)
  line L510 (38.276389, 291.482639) -> (38.170556, 291.553194)
  line L511 (37.958889, 291.059305) -> (38.241111, 291.094583)
  line L512 (38.241111, 291.094583) -> (38.276389, 291.129861)
  line L513 (41.733611, 264.812639) -> (41.557222, 264.847917)
  line L514 (34.572222, 223.36125) -> (34.536944, 223.255417)
  line L515 (38.311667, 242.446528) -> (38.452778, 242.481805)
  line L516 (40.992778, 264.424583) -> (41.133889, 264.63625)
  line L517 (28.433889, 230.381528) -> (27.6225, 230.381528)
  line L518 (27.199167, 289.577639) -> (27.163889, 289.471805)
  line L519 (32.914167, 226.959583) -> (32.878889, 227.030139)
  line L520 (37.817778, 288.166528) -> (37.817778, 289.542361)
  line L521 (34.395833, 291.094583) -> (34.536944, 291.059305)
  line L522 (33.090556, 292.823194) -> (34.29, 291.200417)
  line L523 (32.526111, 292.823194) -> (33.090556, 292.823194)
  line L524 (22.295556, 229.852361) -> (22.189722, 229.852361)
  line L525 (22.189722, 229.852361) -> (22.119167, 229.746528)
  line L526 (17.286111, 223.220139) -> (17.321389, 223.467083)
  line L527 (39.334722, 295.821805) -> (26.3525, 295.821805)
  line L528 (1.446389, 284.391805) -> (1.446389, 282.945417)
  line L529 (14.322778, 295.821805) -> (1.446389, 282.945417)
  line L530 (39.6875, 241.211805) -> (39.405278, 241.14125)
  line L531 (16.898056, 223.149583) -> (17.074444, 223.114305)
  line L532 (16.792222, 223.502361) -> (16.792222, 223.396528)
  line L533 (16.792222, 223.396528) -> (16.792222, 223.325972)
  line L534 (16.792222, 226.994861) -> (16.792222, 223.502361)
  line L535 (32.455556, 238.177917) -> (32.138056, 237.613472)
  line L536 (40.287222, 242.622917) -> (40.357778, 242.234861)
  line L537 (33.408056, 285.555972) -> (33.760833, 285.626528)
  line L538 (33.760833, 285.626528) -> (34.078333, 285.732361)
  line L539 (34.254722, 294.057917) -> (34.219444, 293.84625)
  line L540 (40.3225, 233.239028) -> (40.251944, 233.309583)
  line L541 (40.251944, 233.309583) -> (40.075556, 233.344861)
  line L542 (15.5575, 291.059305) -> (15.204722, 290.953472)
  line L543 (15.204722, 290.953472) -> (14.851944, 290.741805)
  line L544 (30.726944, 289.824583) -> (28.469167, 289.824583)
  line L545 (31.044444, 289.542361) -> (31.009167, 289.683472)
  line L546 (38.664444, 233.344861) -> (40.075556, 233.344861)
  line L547 (34.925, 264.212917) -> (35.454167, 262.378472)
  line L548 (23.106944, 226.53625) -> (23.106944, 226.642083)
  line L549 (23.106944, 226.642083) -> (23.036389, 226.747917)
  line L550 (23.036389, 226.747917) -> (22.930556, 226.889028)
  line L551 (30.973889, 289.365972) -> (30.938611, 289.330694)
  line L552 (31.079722, 295.292639) -> (31.150278, 295.292639)
  line L553 (30.938611, 295.257361) -> (31.079722, 295.292639)
  line L554 (30.868056, 295.186805) -> (30.938611, 295.257361)
  line L555 (31.291389, 295.11625) -> (31.291389, 295.010417)
  line L556 (33.690278, 294.763472) -> (33.831389, 294.728194)
  line L557 (34.007778, 293.52875) -> (33.866667, 293.422917)
  line L558 (39.758056, 234.755972) -> (39.652222, 234.755972)
  line L559 (34.219444, 293.84625) -> (34.113611, 293.634583)
  line L560 (31.044444, 289.542361) -> (31.009167, 289.436528)
  line L561 (23.106944, 226.465694) -> (23.071667, 226.359861)
  line L562 (13.97, 289.471805) -> (13.899444, 289.048472)
  line L563 (20.672778, 295.821805) -> (15.980833, 291.129861)
  line L564 (32.878889, 227.030139) -> (32.843611, 227.135972)
  line L565 (35.348333, 289.648194) -> (35.418889, 289.754028)
  line L566 (28.186944, 289.71875) -> (28.151667, 289.683472)
  line L567 (28.151667, 289.683472) -> (28.116389, 289.577639)
  line L568 (37.676667, 223.290694) -> (37.676667, 223.396528)
  line L569 (39.616944, 244.915972) -> (39.793333, 244.845417)
  line L570 (35.665833, 289.789305) -> (35.736389, 289.754028)
  line L571 (31.150278, 295.292639) -> (31.220833, 295.222083)
  line L572 (38.4175, 244.527917) -> (38.735, 244.810139)
  line L573 (33.619722, 261.179028) -> (33.796111, 261.14375)
  line L574 (33.584444, 261.567083) -> (33.549167, 261.46125)
  line L575 (23.459722, 250.313472) -> (23.530278, 250.313472)
  line L576 (27.6225, 228.970417) -> (27.587222, 228.794028)
  line L577 (35.665833, 291.059305) -> (35.771667, 291.059305)
  line L578 (22.577778, 224.349028) -> (22.577778, 224.137361)
  line L579 (22.577778, 224.137361) -> (22.507222, 223.960972)
  line L580 (22.577778, 225.019305) -> (22.577778, 224.349028)
  line L581 (22.119167, 225.019305) -> (22.577778, 225.019305)
  line L582 (34.642778, 286.614305) -> (34.642778, 287.637361)
  line L583 (34.466389, 286.085139) -> (34.6075, 286.367361)
  line L584 (39.299444, 251.512917) -> (38.523333, 253.065139)
  line L585 (40.040278, 253.100417) -> (39.299444, 251.512917)
  line L586 (32.596667, 235.779028) -> (33.055278, 236.308194)
  line L587 (33.055278, 236.308194) -> (33.478611, 236.872639)
  line L588 (33.478611, 236.872639) -> (33.831389, 237.472361)
  line L589 (33.831389, 237.472361) -> (34.113611, 238.107361)
  line L590 (20.073056, 245.127639) -> (19.755556, 244.527917)
  line L591 (19.755556, 244.527917) -> (19.473333, 243.892917)
  line L592 (19.473333, 243.892917) -> (19.261667, 243.222639)
  line L593 (19.261667, 243.222639) -> (19.120556, 242.552361)
  line L594 (22.471944, 230.416805) -> (22.648333, 230.34625)
  line L595 (22.648333, 230.34625) -> (22.789444, 230.275694)
  line L596 (20.743333, 225.26625) -> (20.778611, 225.548472)
  line L597 (20.778611, 225.548472) -> (20.849167, 225.830694)
  line L598 (30.091944, 294.834028) -> (29.950833, 294.79875)
  line L599 (14.005278, 288.307639) -> (14.181667, 287.954861)
  line L600 (38.241111, 242.340694) -> (38.311667, 242.446528)
  line L601 (39.6875, 244.31625) -> (39.581667, 244.422083)
  line L602 (21.448889, 289.295417) -> (23.459722, 289.295417)
  line L603 (42.474444, 264.777361) -> (42.368611, 264.918472)
  line L604 (30.832778, 291.165139) -> (30.832778, 291.235694)
  line L605 (39.652222, 234.755972) -> (38.664444, 234.755972)
  line L606 (20.531667, 241.77625) -> (20.6375, 242.375972)
  line L607 (39.37, 265.165417) -> (39.440556, 265.306528)
  line L608 (39.440556, 265.306528) -> (39.475833, 265.412361)
  line L609 (37.500278, 261.284861) -> (39.37, 265.165417)
  line L610 (16.086667, 284.885694) -> (21.025556, 284.885694)
  line L611 (24.412222, 247.032639) -> (23.847778, 246.750417)
  line L612 (23.847778, 246.750417) -> (23.318611, 246.432917)
  line L613 (40.251944, 253.20625) -> (40.181389, 253.20625)
  line L614 (40.181389, 253.20625) -> (40.110833, 253.170972)
  line L615 (40.110833, 253.170972) -> (40.040278, 253.100417)
  line L616 (6.385278, 218.034306) -> (11.324167, 218.034306)
  line L617 (36.724167, 218.034306) -> (38.135278, 218.034306)
  line L618 (27.6225, 291.059305) -> (27.551944, 291.059305)
  line L619 (26.176111, 250.313472) -> (26.246667, 250.313472)
  line L620 (26.246667, 250.313472) -> (26.317222, 250.34875)
  line L621 (13.758333, 223.643472) -> (15.804444, 223.643472)
  line L622 (22.366111, 245.656805) -> (22.824722, 246.080139)
  line L623 (37.041667, 261.284861) -> (37.006389, 261.390694)
  line L624 (40.251944, 228.829305) -> (40.3225, 228.899861)
  line L625 (40.3225, 228.899861) -> (40.3225, 228.970417)
  line L626 (39.899167, 228.864583) -> (39.934444, 228.794028)
  line L627 (39.934444, 228.794028) -> (39.969722, 228.75875)
  line L628 (39.969722, 228.75875) -> (40.075556, 228.75875)
  line L629 (28.151667, 224.807639) -> (28.116389, 224.419583)
  line L630 (28.116389, 224.419583) -> (28.010556, 224.137361)
  line L631 (28.151667, 227.030139) -> (28.151667, 224.807639)
  line L632 (30.832778, 294.975139) -> (30.832778, 295.080972)
  line L633 (38.488056, 243.257917) -> (38.382222, 243.434305)
  line L634 (34.148889, 273.490972) -> (34.713333, 275.325417)
  line L635 (40.146111, 243.822361) -> (40.040278, 243.787083)
  line L636 (27.199167, 228.864583) -> (27.199167, 228.970417)
  line L637 (34.254722, 294.057917) -> (34.219444, 294.234305)
  line L638 (34.219444, 294.234305) -> (34.184167, 294.410694)
  line L639 (34.184167, 294.410694) -> (34.043056, 294.587083)
  line L640 (34.043056, 294.587083) -> (33.831389, 294.728194)
  line L641 (33.831389, 294.728194) -> (33.690278, 294.763472)
  line L642 (33.690278, 294.763472) -> (33.513889, 294.763472)
  line L643 (33.513889, 294.763472) -> (32.526111, 294.763472)
  line L644 (32.526111, 294.763472) -> (32.526111, 293.352361)
  line L645 (32.526111, 293.352361) -> (33.443333, 293.352361)
  line L646 (33.443333, 293.352361) -> (33.655, 293.352361)
  line L647 (33.655, 293.352361) -> (33.866667, 293.422917)
  line L648 (33.866667, 293.422917) -> (34.007778, 293.52875)
  line L649 (34.007778, 293.52875) -> (34.113611, 293.634583)
  line L650 (34.113611, 293.634583) -> (34.219444, 293.84625)
  line L651 (34.219444, 293.84625) -> (34.254722, 294.057917)
  line L652 (18.908889, 225.724861) -> (18.803056, 225.58375)
  line L653 (29.280556, 247.032639) -> (29.845, 246.750417)
  line L654 (14.499167, 256.945694) -> (14.181667, 257.01625)
  line L655 (39.264167, 248.020417) -> (39.758056, 246.397639)
  line L656 (39.405278, 265.624028) -> (39.299444, 265.659305)
  line L657 (39.299444, 265.659305) -> (39.228889, 265.694583)
  line L658 (38.981944, 242.975694) -> (38.840833, 243.010972)
  line L659 (34.043056, 226.85375) -> (33.196389, 226.85375)
  line L660 (39.017222, 241.599861) -> (39.123056, 241.599861)
  line L661 (35.348333, 289.507083) -> (35.348333, 289.577639)
  line L662 (28.363333, 223.714028) -> (28.116389, 223.431805)
  line L663 (28.575, 224.066805) -> (28.363333, 223.714028)
  line L664 (27.657778, 223.220139) -> (27.163889, 223.114305)
  line L665 (38.170556, 223.431805) -> (38.170556, 223.36125)
  line L666 (28.116389, 223.431805) -> (27.657778, 223.220139)
  line L667 (29.986111, 250.34875) -> (29.950833, 250.384028)
  line L668 (29.845, 223.643472) -> (31.891111, 223.643472)
  line L669 (24.482778, 285.802917) -> (24.482778, 285.90875)
  line L670 (30.832778, 291.341528) -> (30.832778, 294.975139)
  line L671 (33.090556, 285.59125) -> (32.808333, 285.697083)
  line L672 (32.808333, 285.697083) -> (32.490833, 285.90875)
  line L673 (33.866667, 289.154305) -> (33.655, 289.260139)
  line L674 (33.655, 289.260139) -> (33.443333, 289.295417)
  line L675 (37.676667, 223.396528) -> (37.676667, 223.467083)
  line L676 (25.611667, 224.737083) -> (25.646944, 224.878194)
  line L677 (39.440556, 265.553472) -> (39.405278, 265.624028)
  line L678 (36.477222, 227.241805) -> (36.5125, 227.277083)
  line L679 (25.682222, 224.207917) -> (25.611667, 224.63125)
  line L680 (29.739167, 228.723472) -> (29.668611, 228.75875)
  line L681 (30.127222, 250.313472) -> (30.021389, 250.313472)
  line L682 (27.128611, 285.59125) -> (27.058056, 285.59125)
  line L683 (17.250833, 222.549861) -> (12.735278, 218.034306)
  line L684 (11.324167, 218.034306) -> (15.804444, 222.549861)
  line L685 (11.324167, 218.034306) -> (12.735278, 218.034306)
  line L686 (1.446389, 219.445417) -> (1.446389, 218.034306)
  line L687 (36.5125, 227.277083) -> (36.583056, 227.312361)
  line L688 (27.199167, 231.827917) -> (27.234444, 231.93375)
  line L689 (28.963056, 231.969028) -> (29.033611, 231.898472)
  line L690 (22.895278, 225.548472) -> (23.001111, 225.477917)
  line L691 (16.086667, 223.537639) -> (16.121944, 223.467083)
  line L692 (30.1625, 295.11625) -> (30.1625, 295.045694)
  line L693 (26.211389, 234.085694) -> (26.846389, 234.050417)
  line L694 (26.846389, 234.050417) -> (27.516667, 234.085694)
  line L695 (30.303611, 250.384028) -> (30.233056, 250.313472)
  line L696 (29.915556, 250.560417) -> (29.915556, 252.465417)
  line L697 (29.915556, 252.465417) -> (29.492222, 251.583472)
  line L698 (28.821944, 232.004305) -> (28.963056, 231.969028)
  line L699 (27.340278, 232.004305) -> (27.481389, 232.004305)
  line L700 (33.9725, 241.14125) -> (33.937222, 241.811528)
  line L701 (33.937222, 241.811528) -> (33.831389, 242.446528)
  line L702 (28.680833, 224.701805) -> (28.645556, 224.419583)
  line L703 (28.680833, 227.030139) -> (28.680833, 224.701805)
  line L704 (29.033611, 231.898472) -> (29.068889, 231.792639)
  line L705 (26.634722, 223.220139) -> (26.176111, 223.467083)
  line L706 (29.950833, 250.384028) -> (29.915556, 250.454583)
  line L707 (27.163889, 223.114305) -> (26.634722, 223.220139)
  line L708 (24.235833, 281.745972) -> (19.296944, 281.745972)
  line L709 (27.093333, 289.754028) -> (27.163889, 289.683472)
  line L710 (20.813889, 237.401805) -> (21.166667, 236.872639)
  line L711 (21.166667, 236.872639) -> (21.59, 236.37875)
  line L712 (21.872222, 225.477917) -> (21.942778, 225.513194)
  line L713 (27.446111, 285.944028) -> (27.446111, 285.802917)
  line L714 (42.015833, 262.131528) -> (41.945278, 261.884583)
  line L715 (41.945278, 261.884583) -> (41.874722, 261.77875)
  line L716 (41.874722, 261.77875) -> (41.768889, 261.708194)
  line L717 (34.219444, 288.730972) -> (34.113611, 288.872083)
  line L718 (34.113611, 288.872083) -> (33.866667, 289.154305)
  line L719 (27.446111, 285.802917) -> (27.446111, 285.732361)
  line L720 (43.991389, 295.186805) -> (39.334722, 290.494861)
  line L721 (19.579167, 223.325972) -> (19.579167, 223.396528)
  line L722 (20.6375, 242.375972) -> (20.778611, 243.010972)
  line L723 (29.950833, 253.488472) -> (30.021389, 253.559028)
  line L724 (26.916944, 285.767639) -> (25.964444, 287.390417)
  line L725 (21.59, 236.37875) -> (22.048611, 235.884861)
  line L726 (22.048611, 235.884861) -> (22.577778, 235.461528)
  line L727 (31.785278, 218.034306) -> (36.724167, 218.034306)
  line L728 (36.724167, 218.034306) -> (41.204444, 222.549861)
  line L729 (12.735278, 218.034306) -> (17.674167, 218.034306)
  line L730 (17.674167, 218.034306) -> (22.154444, 222.549861)
  line L731 (16.016111, 223.149583) -> (16.086667, 223.220139)
  line L732 (16.086667, 223.220139) -> (16.121944, 223.255417)
  line L733 (26.916944, 253.594305) -> (26.246667, 253.594305)
  line L734 (27.763611, 252.641805) -> (27.693056, 253.029861)
  line L735 (38.664444, 242.305417) -> (38.664444, 242.199583)
  line L736 (34.113611, 286.790694) -> (34.078333, 286.579028)
  line L737 (33.866667, 293.422917) -> (33.655, 293.352361)
  line L738 (25.0825, 289.789305) -> (25.153056, 289.754028)
  line L739 (32.490833, 285.90875) -> (32.243889, 286.190972)
  line L740 (32.243889, 286.190972) -> (32.032222, 286.473194)
  line L741 (33.443333, 289.295417) -> (33.196389, 289.260139)
  line L742 (33.196389, 289.260139) -> (32.984722, 289.154305)
  line L743 (32.032222, 286.473194) -> (31.891111, 286.790694)
  line L744 (31.891111, 286.790694) -> (31.785278, 287.249305)
  line L745 (37.711944, 293.246528) -> (37.641389, 293.21125)
  line L746 (27.763611, 250.525139) -> (27.763611, 250.454583)
  line L747 (27.763611, 250.454583) -> (27.728333, 250.384028)
  line L748 (27.728333, 250.384028) -> (27.6225, 250.34875)
  line L749 (27.6225, 250.34875) -> (27.551944, 250.313472)
  line L750 (27.551944, 250.313472) -> (27.446111, 250.34875)
  line L751 (27.446111, 250.34875) -> (27.410833, 250.384028)
  line L752 (27.410833, 250.384028) -> (27.375556, 250.419305)
  line L753 (27.375556, 250.419305) -> (26.634722, 251.689305)
  line L754 (26.634722, 251.689305) -> (26.387778, 251.689305)
  line L755 (26.387778, 251.689305) -> (26.387778, 250.560417)
  line L756 (26.387778, 250.560417) -> (26.3525, 250.384028)
  line L757 (26.3525, 250.384028) -> (26.317222, 250.34875)
  line L758 (26.317222, 250.34875) -> (26.246667, 250.313472)
  line L759 (26.246667, 250.313472) -> (26.176111, 250.313472)
  line L760 (26.176111, 250.313472) -> (26.070278, 250.313472)
  line L761 (26.070278, 250.313472) -> (25.999722, 250.384028)
  line L762 (25.999722, 250.384028) -> (25.964444, 250.419305)
  line L763 (25.964444, 250.419305) -> (25.964444, 250.454583)
  line L764 (25.964444, 250.454583) -> (25.964444, 250.595694)
  line L765 (25.964444, 250.595694) -> (25.964444, 253.312083)
  line L766 (25.964444, 253.312083) -> (25.964444, 253.417917)
  line L767 (25.964444, 253.417917) -> (25.999722, 253.52375)
  line L768 (25.999722, 253.52375) -> (26.105556, 253.594305)
  line L769 (26.105556, 253.594305) -> (26.246667, 253.594305)
  line L770 (26.246667, 253.594305) -> (26.916944, 253.594305)
  line L771 (26.916944, 253.594305) -> (27.199167, 253.559028)
  line L772 (27.199167, 253.559028) -> (27.481389, 253.382639)
  line L773 (27.481389, 253.382639) -> (27.693056, 253.029861)
  line L774 (27.693056, 253.029861) -> (27.763611, 252.641805)
  line L775 (27.763611, 252.641805) -> (27.728333, 252.394861)
  line L776 (27.728333, 252.394861) -> (27.6225, 252.147917)
  line L777 (27.6225, 252.147917) -> (27.446111, 251.865694)
  line L778 (27.446111, 251.865694) -> (27.128611, 251.724583)
  line L779 (27.128611, 251.724583) -> (27.093333, 251.689305)
  line L780 (27.093333, 251.689305) -> (27.693056, 250.701528)
  line L781 (27.693056, 250.701528) -> (27.693056, 250.66625)
  line L782 (27.693056, 250.66625) -> (27.728333, 250.595694)
  line L783 (27.728333, 250.595694) -> (27.763611, 250.560417)
  line L784 (27.763611, 250.560417) -> (27.763611, 250.525139)
  line L785 (30.374167, 246.432917) -> (29.845, 246.750417)
  line L786 (29.845, 246.750417) -> (29.280556, 247.032639)
  line L787 (38.135278, 253.100417) -> (38.205833, 253.170972)
  line L788 (21.025556, 284.885694) -> (17.885833, 281.745972)
  line L789 (12.594167, 223.431805) -> (12.523611, 223.220139)
  line L790 (23.777222, 285.979305) -> (23.636111, 286.085139)
  line L791 (30.268333, 253.559028) -> (30.197778, 253.594305)
  line L792 (30.197778, 253.594305) -> (30.127222, 253.594305)
  line L793 (30.374167, 246.432917) -> (30.868056, 246.080139)
  line L794 (13.758333, 225.26625) -> (15.204722, 225.26625)
  line L795 (13.758333, 223.643472) -> (13.758333, 225.26625)
  line L796 (15.804444, 223.643472) -> (13.758333, 223.643472)
  line L797 (29.21, 293.175972) -> (27.798889, 293.175972)
  line L798 (24.306389, 248.584861) -> (23.636111, 248.337917)
  line L799 (23.636111, 248.337917) -> (23.036389, 248.020417)
  line L800 (23.036389, 248.020417) -> (22.436667, 247.667639)
  line L801 (34.078333, 286.579028) -> (34.043056, 286.402639)